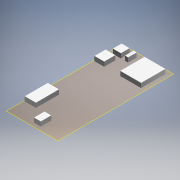
# Autodesk Inventor part: 02_Anschluss
Saved by Autodesk Inventor 2016 (Build 200138000, 138)
## iProperties
Created: 2016-11-08
Part Number: 02_Anschluss
Material: Generisch
Document SubType Name: Modeling
Designer: Bene
Density: 1 g/cm^3
Appearance: Chrom - poliert
Author: Bene
Autodesk Inventor part; units mm, degrees
ref_plane "YZ Plane" through (0, 0, 0) normal (1, 0, 0) x (0, 1, 0)
ref_plane "XZ Plane" through (0, 0, 0) normal (0, 1, 0) x (-1, 0, 0)
ref_plane "XY Plane" through (0, 0, 0) normal (0, 0, 1) x (1, 0, 0)
ref_plane "Arbeitsebene1" through (0, 2, 0) normal (0, 0, 1) x (1, 0, 0)
sketch "Skizze1" plane through (0, 2, 0) normal (0, 0, 1) x (1, 0, 0)
  circle A0 centre (-20.2101, 32.0775) radius 3.5 projected
  circle A1 centre (16.2899, -69.9225) radius 3.5 projected
  circle A2 centre (27.7899, 29.0775) radius 1.5 projected
  circle A3 centre (-1.7101, -53.9225) radius 1.5 projected
  line L0 (-11.7101, -74.9225) -> (30.2899, -74.9225) projected
  line L1 (30.2899, -74.9225) -> (30.2899, 66.0775) projected
  line L2 (30.2899, 66.0775) -> (-32.7101, 66.0775) projected
  line L3 (-32.7101, 66.0775) -> (-32.7101, -53.9225) projected
  line L4 (-32.7101, -53.9225) -> (-11.7101, -74.9225) projected
  line L5 (27.7899, 69.6886) -> (-0.2101, 69.6886)
  line L6 (-0.2101, 69.6886) -> (-0.2101, 35.0775)
  line L7 (-0.2101, 35.0775) -> (27.7899, 35.0775)
  line L8 (27.7899, 35.0775) -> (27.7899, 69.6886)
  line L9 (-10.5357, 69.6886) -> (-14.6669, 69.6886)
  line L10 (-14.6669, 69.6886) -> (-14.6669, 57.9834)
  line L11 (-14.6669, 57.9834) -> (-10.5357, 57.9834)
  line L12 (-10.5357, 57.9834) -> (-10.5357, 69.6886)
  line L13 (-20.2101, 69.6886) -> (-30.9624, 69.6886)
  line L14 (-30.9624, 69.6886) -> (-30.9624, 57.9834)
  line L15 (-30.9624, 57.9834) -> (-20.2101, 57.9834)
  line L16 (-20.2101, 57.9834) -> (-20.2101, 69.6886)
  line L17 (-21.7101, 50.0775) -> (-34.7101, 50.0775)
  line L18 (-34.7101, 50.0775) -> (-34.7101, 35.0775)
  line L19 (-34.7101, 35.0775) -> (-21.7101, 35.0775)
  line L20 (-21.7101, 35.0775) -> (-21.7101, 50.0775)
  line L21 (-19.7101, -27.4225) -> (-34.7101, -27.4225)
  line L22 (-34.7101, -27.4225) -> (-34.7101, -58.4225)
  line L23 (-34.7101, -58.4225) -> (-19.7101, -58.4225)
  line L24 (-19.7101, -58.4225) -> (-19.7101, -27.4225)
  line L25 (-3.7101, -62.9225) -> (5.2899, -62.9225)
  line L26 (5.2899, -62.9225) -> (5.2899, -76.9225)
  line L27 (5.2899, -76.9225) -> (-3.7101, -76.9225)
  line L28 (-3.7101, -76.9225) -> (-3.7101, -62.9225)
  point P0 (0, -2)
  dimension "d0" = 16
  dimension "d1" = 15
  dimension "d2" = 2
  dimension "d3" = 13
  dimension "d4" = 16.5
  dimension "d5" = 0
  dimension "d6" = 15
  dimension "d7" = 31
  dimension "d8" = 25
  dimension "d9" = 9
  dimension "d10" = 14
  dimension "d11" = 2
  constraints: 48 end point, 12 parallel, 6 horizontal, 6 perpendicular, 4 point on line
  measures "d0" distance from line of L17 L2.end
  measures "d1" distance between parallel lines of L17 L19
  measures "d2" distance between parallel lines of L18 L3
  measures "d3" distance between parallel lines of L18 L20
  measures "d4" distance between parallel lines of L23 L0
  measures "d5" distance between parallel lines of L18 L22
  measures "d6" distance between parallel lines of L22 L24
  measures "d7" distance between parallel lines of L21 L23
  measures "d8" distance between parallel lines of L26 L1
  measures "d9" distance between parallel lines of L28 L26
  measures "d10" distance between parallel lines of L25 L27
  measures "d11" distance between parallel lines of L27 L0
extrude "Extrusion1" add sketch "Skizze1" along normal blind 6 contours L20 L19 A0 | A0 L19 L3 L17 L20 | L19 L18 L17 L3 | L21 L24 L23 L4 L3 | L3 L4 L23 L22 L21 | L14 L13 L16 L2 | L2 L16 L15 L14 | L10 L9 L12 L2 | L2 L12 L11 L10 | L28 L25 L26 L0 | L0 L26 L27 L28 | L6 L5 L8 L2 | L2 L8 L7 L6 picked at (-21.8789, 35.0966)
ref_plane "Arbeitsebene2" through (-6.2387, 2, -1) normal (0, 0, -1) x (-1, 0, 0)
sketch "Skizze2" plane through (-6.2387, 2, -1) normal (0, 0, -1) x (-1, 0, 0)
  circle A0 centre (13.9714, 32.0775) radius 3.5 projected
  circle A1 centre (-22.5286, -69.9225) radius 3.5 projected
  circle A2 centre (-34.0286, 29.0775) radius 1.5 projected
  circle A3 centre (-4.5286, -53.9225) radius 1.5 projected
  line L0 (-36.5286, -74.9225) -> (5.4714, -74.9225) projected
  line L1 (5.4714, -74.9225) -> (26.4714, -53.9225) projected
  line L2 (26.4714, -53.9225) -> (26.4714, 66.0775) projected
  line L3 (26.4714, 66.0775) -> (-36.5286, 66.0775) projected
  line L4 (-36.5286, 66.0775) -> (-36.5286, -74.9225) projected
  circle A4 centre (11.4714, -48.9225) radius 4.0524
  point P0 (-6.2387, -2)
  dimension "d14" = 15
  dimension "d15" = 26
  constraints: 1 centre point
  measures "d14" distance from line of A4.centre L2
  measures "d15" distance from line of A4.centre L0
extrude "Extrusion2" add sketch "Skizze2" along normal blind 3 contours A4
